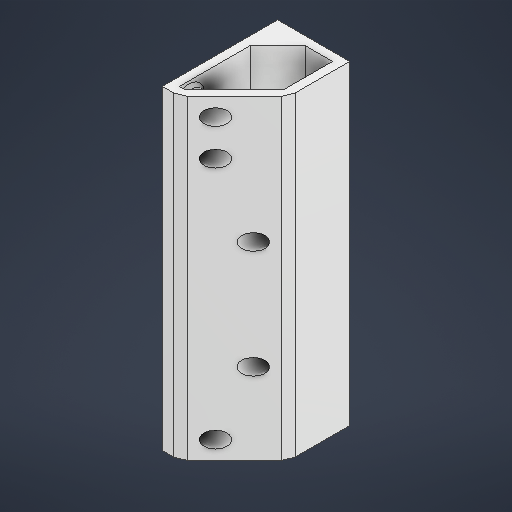
# Autodesk Inventor part: CNC-031-BackCover1
Saved by Autodesk Inventor 2026.2 (Build 302298000, 298)
## iProperties
Created: 2026-06-28
Part Number: CNC-031-BackCover1
Material: ABS Plastic
Document SubType Name: Modeling
Designer: Kenji
Density: 1.06 g/cm^3
Appearance: Smooth - White
Author: Kenji
Autodesk Inventor part; units mm, degrees
ref_plane "YZ Plane" through (0, 0, 0) normal (1, 0, 0) x (0, 1, 0)
ref_plane "XZ Plane" through (0, 0, 0) normal (0, 1, 0) x (-1, 0, 0)
ref_plane "XY Plane" through (0, 0, 0) normal (0, 0, 1) x (1, 0, 0)
sketch "Sketch1" plane through (0, 0, 0) normal (0, 1, 0) x (-1, 0, 0)
  line L0 (40, 10) -> (40, -10)
  line L1 (0, -54) -> (20, -54)
  line L2 (0, -54) -> (0, -20.475)
  line L3 (40, 10) -> (30.475, 10)
  line L4 (30.475, 10) -> (0, -20.475)
  line L5 (40, -10) -> (34.7217, -10)
  line L6 (34.7217, -10) -> (20, -24.7217)
  line L7 (20, -24.7217) -> (20, -54)
  point P0 (0, 0)
  point P1 (40, 0)
  dimension "d0" = 20
  dimension "d1" = 40
  dimension "d2" = 44
  dimension "d3" = 9.525
  dimension "d4" = 135
  dimension "d5" = 17.145
  constraints: 16 end point, 3 horizontal, 3 vertical, 1 horizontal alignment, 1 midpoint, 1 parallel, 1 perpendicular, 1 point on line, 1 vertical alignment
  measures "d0" distance of L0.start L0.end
  measures "d1" distance from line of L0 point (0, 0)
  measures "d2" distance from line of L1 L0.end
  measures "d3" distance of L3.end L0.start
  measures "d4" angle of L4 L3
  measures "d5" distance between parallel lines of L4 L6
extrude "Extrusion1" add sketch "Sketch1" along normal blind 175
sketch "Sketch2" plane through (0, 175, 0) normal (0, 1, 0) x (1, 0, 0)
  line L0 (0, 20.475) -> (0, 54) projected
  line L1 (0, 54) -> (-20, 54) projected
  line L2 (-20, 54) -> (-20, 24.7217) projected
  line L3 (-20, 24.7217) -> (-34.7217, 10) projected
  line L4 (-34.7217, 10) -> (-40, 10) projected
  line L5 (-40, 10) -> (-40, -10) projected
  line L6 (-40, -10) -> (-30.475, -10) projected
  line L7 (-30.475, -10) -> (0, 20.475) projected
  line L8 (-15.2375, 49.2375) -> (-4.7625, 49.2375)
  line L9 (-4.7625, 49.2375) -> (-4.7625, 22.4477)
  line L10 (-4.7625, 22.4477) -> (-32.4477, -5.2375)
  line L11 (-32.4477, -5.2375) -> (-35.2375, -5.2375)
  line L12 (-35.2375, -5.2375) -> (-35.2375, 5.2375)
  line L13 (-35.2375, 5.2375) -> (-35.2375, 10)
  line L14 (-15.2375, 49.2375) -> (-20, 49.2375)
  point P0 (0, 0)
  dimension "d9" = 4.7625
  constraints: 14 end point, 2 perpendicular, 2 point on line, 4 other
  measures "d9" distance between parallel lines of L1 L14
extrude "Extrusion2" cut sketch "Sketch2" against normal through all contours L14 L8 L9 L10 L11 L12 L13 L4 L3 L2
sketch "Sketch3" plane through (-40, 0, -10) normal (-1, 0, 0) x (0, 0, 1)
  circle A0 centre (10, 165) radius 2.63
  line L0 (0, 175) -> (20, 175) projected
  line L1 (20, 0) -> (20, 175) projected
  circle A1 centre (10, 145) radius 2.63
  circle A2 centre (10, 125) radius 2.63 construction
  circle A3 centre (10, 105) radius 2.63 construction
  circle A4 centre (10, 85) radius 2.63
  circle A5 centre (10, 65) radius 2.63
  circle A6 centre (10, 45) radius 2.63 construction
  circle A7 centre (10, 25) radius 2.63 construction
  circle A8 centre (10, 5) radius 2.63 construction
  circle A9 centre (10, -15) radius 2.63
  point P0 (10, 0)
  dimension "d12" = 5.26
  dimension "d13" = 10
  dimension "d14" = 10
  dimension "d17" = 20
  constraints: 10 centre point, 1 vertical, 18 other
  measures "d12" diameter of A0
  measures "d13" distance from line of A0.centre L0
  measures "d14" distance from line of L1 A0.centre
  measures "d17" distance of A0.centre A1.centre
extrude "Extrusion3" cut sketch "Sketch3" against normal blind 25.4
sketch "Sketch4" plane through (-35.2375, 175, 5.2375) normal (1, 0, 0) x (0, 0, -1)
  circle A0 centre (5.2375, -90) radius 2.63 projected
  circle A1 centre (5.2375, -110) radius 2.63 projected
  circle A2 centre (5.2375, -30) radius 2.63 projected
  circle A3 centre (5.2375, -10) radius 2.63 projected
  line L0 (15.2375, -175) -> (0, -175) projected
  line L1 (15.2375, 0) -> (15.2375, -175) projected
  line L2 (0, 0) -> (15.2375, 0) projected
  line L3 (0, 0) -> (0, -175) projected
  circle A4 centre (5.2375, -10) radius 7
  circle A5 centre (5.2375, -30) radius 7
  circle A6 centre (5.2375, -90) radius 7
  circle A7 centre (5.2375, -110) radius 2.63 projected
  circle A8 centre (5.2375, -110) radius 7
  point P0 (5.2375, -175)
  dimension "d24" = 14
  constraints: 4 centre point, 4 coincident, 3 equal radius
  measures "d24" diameter of A4
extrude "Extrusion4" add sketch "Sketch4" along normal up to surface contours A8 L3 | L3 A8 | A4 L3 | L3 A4 | A6 L3 | L3 A6 | A5 L3 | L3 A5 surface through (-4.7625, 175, -22.4477) normal (0.7071068, 0, 0.7071068)
sketch "Sketch5" plane through (0, 0, -20.475) normal (1, 0, 0) x (0, 0, -1)
  circle A0 centre (-20.475, 65) radius 2.63 projected
  circle A1 centre (-20.475, 85) radius 2.63 projected
  circle A2 centre (-20.475, 145) radius 2.63 projected
  circle A3 centre (-20.475, 165) radius 2.63 projected
  circle A4 centre (-20.475, 165) radius 4.5
  circle A5 centre (-20.475, 145) radius 4.5
  circle A6 centre (-20.475, 85) radius 4.5
  circle A7 centre (-20.475, 65) radius 4.5
  circle A8 centre (-20.475, 10) radius 4.5
  point P0 (-20.475, 0)
  dimension "d27" = 9
  constraints: 5 centre point, 5 coincident, 4 equal radius
  measures "d27" diameter of A4
extrude "Extrusion5" cut sketch "Sketch5" against normal blind 38.2298
chamfer "Chamfer1" distance 1.5875 angle 45 12 edges at (-35.2375, 165, -7) (-24.7265, 171.5446, -2.4837) (-24.7265, 158.4554, -2.4837) (-35.2375, 145, -7) (-24.7265, 151.5446, -2.4837) (-24.7265, 138.4554, -2.4837) (-24.7265, 78.4554, -2.4837) (-24.7265, 91.5446, -2.4837) (-24.7265, 58.4554, -2.4837) (-24.7265, 71.5446, -2.4837) (-35.2375, 65, -7) (-35.2375, 85, -7)
chamfer "Chamfer3" distance 3.175 angle 45 2 edges at (-30.475, 87.5, 10) (0, 87.5, -20.475)
sketch "Sketch6" plane through (0, 175, 0) normal (0, 1, 0) x (1, 0, 0)
  line L0 (0, 54) -> (-20, 54) projected
  line L1 (-20, 54) -> (-40, 54)
  line L2 (-40, 10) -> (-40, -10) projected
  line L3 (-40, 54) -> (-40, 10)
  line L4 (-20, 54) -> (-20, 49.2375) projected
  line L5 (-35.2375, 10) -> (-35.2375, -5.2375) projected
  line L6 (-20, 49.2375) -> (-35.2375, 34)
  line L7 (-35.2375, 34) -> (-35.2375, 10)
  line L8 (-20, 49.2375) -> (-4.7625, 49.2375) projected
  line L9 (-35.2375, 10) -> (-40, 10)
  point P0 (0, 0)
  dimension "d39" = 135
  constraints: 10 end point, 2 horizontal, 2 vertical
  measures "d39" angle of L8 L6
extrude "Extrusion6" add sketch "Sketch6" against normal up to surface (175 mm away)
sketch "Sketch7" plane through (-35.2375, 0, 5.2375) normal (1, 0, 0) x (0, 0, -1)
  circle A0 centre (5.2375, 10) radius 4.5 projected
  circle A1 centre (5.2375, 10) radius 7
  point P0 (5.2375, 0)
  dimension "d42" = 14
  constraints: 1 centre point, 1 coincident
  measures "d42" diameter of A1
extrude "Extrusion7" add sketch "Sketch7" along normal up to surface surface through (-4.7625, 175, -22.4477) normal (0.7071068, 0, 0.7071068)
sketch "Sketch8" plane through (-35.2375, 10, 0) normal (1, 0, 0) x (0, -1, 0)
  circle A0 centre (0, 0) radius 2.63
  point P0 (10, 0)
  dimension "d45" = 5.26
  constraints: 1 centre point, 1 coincident, 1 other
  measures "d45" diameter of A0
extrude "Extrusion8" cut sketch "Sketch8" against normal through all
sketch "Sketch9" plane through (-40, 0, 10) normal (0, 0, 1) x (1, 0, 0)
  circle A0 centre (30, 30) radius 4.5
  circle A1 centre (19.525, 10) radius 4.5 projected
  line L0 (40, 0) -> (40, 175) projected
  circle A2 centre (19.525, 65) radius 4.5 projected
  circle A3 centre (19.525, 85) radius 4.5 projected
  circle A4 centre (19.525, 145) radius 4.5 projected
  circle A5 centre (19.525, 165) radius 4.5 projected
  circle A6 centre (30, 45) radius 4.5
  circle A7 centre (30, 105) radius 4.5
  circle A8 centre (30, 125) radius 4.5
  dimension "d48" = 10
  dimension "d49" = 20
  dimension "d50" = 20
  dimension "d51" = 20
  dimension "d52" = 20
  constraints: 4 centre point, 4 equal radius, 3 vertical alignment
  measures "d48" distance from line of A0.centre L0
  measures "d49" vertical distance of A0.centre A1.centre
  measures "d50" vertical distance of A2.centre A6.centre
  measures "d51" vertical distance of A7.centre A3.centre
  measures "d52" vertical distance of A4.centre A8.centre
extrude "Extrusion9" cut sketch "Sketch9" against normal blind 62.2328 contours A0 | A6 | A7 | A8
sketch "Sketch10" plane through (-4.7625, 0, -49.2375) normal (0, 0, 1) x (1, 0, 0)
  circle A0 centre (-5.2375, 30) radius 4.5 projected
  circle A1 centre (-5.2375, 45) radius 4.5 projected
  circle A2 centre (-5.2375, 105) radius 4.5 projected
  circle A3 centre (-5.2375, 125) radius 4.5 projected
  circle A4 centre (-5.2375, 125) radius 7
  circle A5 centre (-5.2375, 105) radius 7
  circle A6 centre (-5.2375, 45) radius 7
  circle A7 centre (-5.2375, 30) radius 7
  point P0 (4.7625, 0)
  dimension "d55" = 14
  constraints: 4 centre point, 4 coincident, 3 equal radius
  measures "d55" diameter of A4
extrude "Extrusion10" add sketch "Sketch10" along normal up to surface surface through (-4.7625, 175, -22.4477) normal (0.7071068, 0, 0.7071068)
sketch "Sketch11" plane through (-10, 125, -49.2375) normal (0, 0, 1) x (0, 1, 0)
  circle A0 centre (0, -95) radius 4.5 projected
  circle A1 centre (0, -80) radius 4.5 projected
  circle A2 centre (0, -20) radius 4.5 projected
  circle A3 centre (0, 0) radius 4.5 projected
  circle A4 centre (0, -20) radius 2.63
  circle A5 centre (0, 0) radius 2.63
  circle A6 centre (0, -80) radius 2.63
  circle A7 centre (0, -95) radius 2.63
  point P0 (-125, -10)
  dimension "d58" = 5.26
  constraints: 4 centre point, 4 coincident, 3 equal radius
  measures "d58" diameter of A4
extrude "Extrusion11" cut sketch "Sketch11" against normal blind 25.4 contours A4 | A5 | A6 | A7
sketch "Sketch12" plane through (-40, 175, -54) normal (-1, 0, 0) x (0, 0, 1)
  circle A0 centre (54, -90) radius 2.63 projected
  circle A1 centre (54, -110) radius 2.63 projected
  circle A2 centre (54, -90) radius 2.63 projected
  circle A3 centre (54, -90) radius 4.5
  circle A4 centre (54, -110) radius 4.5 projected
  circle A5 centre (54, -110) radius 4.5
  point P0 (54, -175)
  constraints: 2 centre point, 2 coincident, 2 equal radius
extrude "Extrusion12" add sketch "Sketch12" against normal up to surface contours A0 | A1 | A3 | A4 surface through (-30.475, 0, 10) normal (0.7071068, 0, 0.7071068)
sketch "Sketch13" plane through (0, 0, -54) normal (0, 0, -1) x (-1, 0, 0)
  circle A0 centre (10, 125) radius 2.63 projected
  circle A1 centre (10, 30) radius 2.63 projected
  circle A2 centre (10, 30) radius 2.63 projected
  circle A3 centre (10, 30) radius 4.5
  circle A4 centre (10, 125) radius 4.5 projected
  circle A5 centre (10, 125) radius 4.5
  circle A6 centre (10, 30) radius 4.5 projected
  point P0 (0, 0)
  constraints: 2 centre point, 2 coincident, 2 equal radius
extrude "Extrusion13" add sketch "Sketch13" against normal up to surface contours A0 | A1 | A3 | A4 surface through (-30.475, 0, 10) normal (0.7071068, 0, 0.7071068)
equation "\"d50\" = d49"
equation "\"d51\" = d49"
equation "\"d52\" = d51"
body "Solid1"
